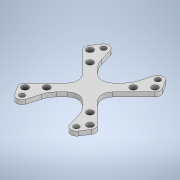
# Autodesk Inventor part: 2030fermto
Saved by Autodesk Inventor 2020.2 (Build 242310000, 310)
## iProperties
Created: 2025-11-08
Part Number: 2030fermto
Material: Типовые
Document SubType Name: Modeling
Designer: pickaxe
Density: 1 g/cm^3
Appearance: По умолчанию
Author: pickaxe
Autodesk Inventor part; units mm, degrees
ref_plane "YZ Plane" through (0, 0, 0) normal (1, 0, 0) x (0, 1, 0)
ref_plane "XZ Plane" through (0, 0, 0) normal (0, 1, 0) x (-1, 0, 0)
ref_plane "XY Plane" through (0, 0, 0) normal (0, 0, 1) x (1, 0, 0)
sketch "Эскиз1" plane through (0, 0, 0) normal (0, 1, 0) x (-1, 0, 0)
  circle A0 centre (12.55, 18.8) radius 1.25
  circle A1 centre (-12.55, 18.8) radius 1.25
  circle A2 centre (-12.55, -18.8) radius 1.25
  circle A3 centre (12.55, -18.8) radius 1.25
  circle A4 centre (15, -15) radius 1.5
  circle A5 centre (15, 15) radius 1.5
  circle A6 centre (10, 10) radius 1.5
  circle A7 centre (10, -10) radius 1.5
  circle A8 centre (-10, 10) radius 1.5
  circle A9 centre (-10, -10) radius 1.5
  circle A10 centre (-15, -15) radius 1.5
  circle A11 centre (-15, 15) radius 1.5
  arc A12 (16.7678, 13.2322) -> (17.1011, 16.3547) centre (15, 15) ccw
  arc A13 (-16.7678, -13.2322) -> (-17.1011, -16.3547) centre (-15, -15) ccw
  arc A14 (17.1011, -16.3547) -> (16.7678, -13.2322) centre (15, -15) ccw
  arc A15 (-17.1011, 16.3547) -> (-16.7678, 13.2322) centre (-15, 15) ccw
  line L0 (16.7678, -13.2322) -> (7.0711, -3.5355)
  line L1 (-3.5355, 7.0711) -> (-5.9595, 9.4951)
  line L2 (-5.9595, -9.4951) -> (-3.5355, -7.0711)
  line L3 (7.0711, 3.5355) -> (16.7678, 13.2322)
  line L4 (5.9595, 9.4951) -> (3.5355, 7.0711)
  line L5 (-7.0711, -3.5355) -> (-16.7678, -13.2322)
  line L6 (-16.7678, 13.2322) -> (-7.0711, 3.5355)
  line L7 (3.5355, -7.0711) -> (5.9595, -9.4951)
  line L8 (10.1488, 19.4958) -> (8.4933, 13.7829)
  arc A16 (14.6511, 20.1547) -> (10.1488, 19.4958) centre (12.55, 18.8) ccw
  line L9 (10, -10) -> (12.55, -18.8) construction
  line L10 (8.4933, -13.7829) -> (10.1488, -19.4958)
  arc A17 (10.1488, -19.4958) -> (14.6511, -20.1547) centre (12.55, -18.8) ccw
  line L11 (-10.1488, -19.4958) -> (-8.4933, -13.7829)
  arc A18 (-14.6511, -20.1547) -> (-10.1488, -19.4958) centre (-12.55, -18.8) ccw
  line L12 (-8.4933, 13.7829) -> (-10.1488, 19.4958)
  arc A19 (-10.1488, 19.4958) -> (-14.6511, 20.1547) centre (-12.55, 18.8) ccw
  line L13 (10, 10) -> (10.4175, 11.4407) construction
  line L14 (12.2021, 17.5994) -> (12.55, 18.8) construction
  line L15 (12.55, 18.8) -> (15, 15) construction
  line L16 (17.1011, 16.3547) -> (14.6511, 20.1547)
  arc A20 (14.6511, 20.1547) -> (10.1488, 19.4958) centre (12.55, 18.8) ccw
  arc A21 (16.7678, 13.2322) -> (17.1011, 16.3547) centre (15, 15) ccw
  line L17 (15, -15) -> (12.55, -18.8) construction
  line L18 (11.8055, -15.3411) -> (11.6276, -15.617)
  line L19 (14.6511, -20.1547) -> (17.1011, -16.3547)
  arc A22 (17.1011, -16.3547) -> (16.7678, -13.2322) centre (15, -15) ccw
  arc A23 (10.1488, -19.4958) -> (14.6511, -20.1547) centre (12.55, -18.8) ccw
  line L20 (-12.55, -18.8) -> (-15, -15) construction
  line L21 (-17.1011, -16.3547) -> (-14.6511, -20.1547)
  arc A24 (-14.6511, -20.1547) -> (-10.1488, -19.4958) centre (-12.55, -18.8) ccw
  arc A25 (-16.7678, -13.2322) -> (-17.1011, -16.3547) centre (-15, -15) ccw
  line L22 (-15, 15) -> (-12.55, 18.8) construction
  line L23 (-14.6511, 20.1547) -> (-17.1011, 16.3547)
  arc A26 (-17.1011, 16.3547) -> (-16.7678, 13.2322) centre (-15, 15) ccw
  arc A27 (-10.1488, 19.4958) -> (-14.6511, 20.1547) centre (-12.55, 18.8) ccw
  arc A28 (7.0711, 3.5355) -> (7.0711, -3.5355) centre (10.6066, 0) ccw
  arc A29 (-3.5355, 7.0711) -> (3.5355, 7.0711) centre (0, 10.6066) ccw
  arc A30 (3.5355, -7.0711) -> (-3.5355, -7.0711) centre (0, -10.6066) ccw
  arc A31 (-7.0711, -3.5355) -> (-7.0711, 3.5355) centre (-10.6066, 0) ccw
  arc A32 (5.9595, 9.4951) -> (8.4933, 13.7829) centre (-1.1115, 16.5661) ccw
  arc A33 (-8.4933, 13.7829) -> (-5.9595, 9.4951) centre (1.1115, 16.5661) ccw
  arc A34 (-5.9595, -9.4951) -> (-8.4933, -13.7829) centre (1.1115, -16.5661) ccw
  arc A35 (8.4933, -13.7829) -> (5.9595, -9.4951) centre (-1.1115, -16.5661) ccw
  point P0 (0, 0)
  point P1 (0, 0)
  point P2 (0, 0)
  point P3 (11.275, 14.4)
  point P4 (11.275, -14.4)
  point P5 (-11.275, -14.4)
  point P6 (-11.275, 14.4)
  point P7 (13.775, 16.9)
  point P8 (13.775, -16.9)
  point P9 (-13.775, -16.9)
  point P10 (-13.775, 16.9)
  dimension "d12" = 3
  dimension "d7" = 2.5
  dimension "d8" = 2.5
  dimension "d9" = 2.5
  dimension "d10" = 3
  dimension "d11" = 3
  dimension "d13" = 3
  dimension "d14" = 3
  dimension "d15" = 3
  dimension "d16" = 3
  dimension "d17" = 3
  dimension "d21" = 5
  dimension "d24" = 5
  dimension "d25" = 5
  dimension "d26" = 5
  dimension "d27" = 5
  dimension "d28" = 5
  dimension "d29" = 10
  constraints: 58 end point, 48 point on circle, 46 tangent, 34 centre point, 10 equal radius, 10 parallel, 5 midpoint, 2 point on line, 6 other
  measures "d7" diameter of A1
  measures "d8" diameter of A2
  measures "d9" diameter of A3
  measures "d10" diameter of A4
  measures "d11" diameter of A5
  measures "d13" diameter of A7
  measures "d14" diameter of A8
  measures "d15" diameter of A9
  measures "d16" diameter of A10
  measures "d17" diameter of A11
  measures "d21" diameter of A17
  measures "d24" diameter of A21
  measures "d25" diameter of A23
  measures "d26" diameter of A25
  measures "d27" diameter of A27
  measures "d28" radius of A28
  measures "d29" radius of A32
extrude "Выдавливание1" add sketch "Эскиз1" along normal blind 2
